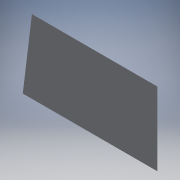
# Autodesk Inventor part: Grundstück
Saved by Autodesk Inventor 2017 (Build 210142000, 142)
## iProperties
Created: 2017-05-10
Part Number: Grundstück
Material: Generic
Document SubType Name: Modeling
Designer: Fake
Density: 1 g/cm^3
Appearance: Default
Author: Fake
Autodesk Inventor part; units mm, degrees
ref_plane "YZ Plane" through (0, 0, 0) normal (1, 0, 0) x (0, 1, 0)
ref_plane "XZ Plane" through (0, 0, 0) normal (0, 1, 0) x (-1, 0, 0)
ref_plane "XY Plane" through (0, 0, 0) normal (0, 0, 1) x (1, 0, 0)
sketch "Skizze1" plane through (0, 0, 0) normal (0, 1, 0) x (-1, 0, 0)
  line L0 (41000, 24000) -> (0, 24000)
  line L1 (0, 24000) -> (0, 0)
  line L2 (0, 0) -> (44000, 0)
  line L3 (44000, 0) -> (41000, 24000)
  line L4 (52800, 0) -> (-8800, 0) projected
  line L5 (0, -4800) -> (0, 28800) projected
  dimension "d2" = 44000
  dimension "d3" = 24000
  dimension "d4" = 41000
  constraints: 9 end point, 2 perpendicular, 2 point on line, 1 horizontal
  measures "d2" distance of L1.end L2.end
  measures "d3" distance of L0.end L1.end
  measures "d4" distance of L0.start L0.end
extrude "Extrusion1" add sketch "Skizze1" against normal blind 1
